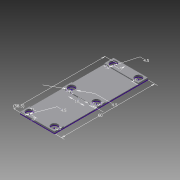
# Autodesk Inventor part: FoldLink
Saved by Autodesk Inventor 2014 SP1 (Build 180222100, 222)
## iProperties
Created: 2015-03-29
Part Number: FoldLink
Material: Generic
Document SubType Name: Modeling
Designer: Erin
Density: 1 g/cm^3
Appearance: Default
Author: Erin
Autodesk Inventor part; units mm, degrees
ref_plane "YZ Plane" through (0, 0, 0) normal (1, 0, 0) x (0, 1, 0)
ref_plane "XZ Plane" through (0, 0, 0) normal (0, 1, 0) x (-1, 0, 0)
ref_plane "XY Plane" through (0, 0, 0) normal (0, 0, 1) x (1, 0, 0)
sketch "Sketch1" plane through (0, 0, 0) normal (0, 0, 1) x (1, 0, 0)
  line L0 (-11, -30) -> (11, -30)
  line L1 (11, -30) -> (11, 30)
  line L2 (11, 30) -> (-11, 30)
  line L3 (-11, 30) -> (-11, -30)
  circle A0 centre (-8, 0) radius 2.25
  line L4 (-5, 30) -> (-5, -30) construction
  line L5 (5, 30) -> (5, -30) construction
  line L6 (0, 30) -> (0, -30) construction
  circle A1 centre (-8, 27) radius 2.25
  circle A2 centre (-8, -27) radius 2.25
  circle A3 centre (8, -27) radius 2.25
  circle A4 centre (8, 0) radius 2.25
  circle A5 centre (8, 27) radius 2.25
  line L7 (-11, 0) -> (11, 0) construction
  line L8 (-11, 30) -> (11, 30)
  line L9 (11, 30) -> (11, 24)
  line L10 (11, 24) -> (-11, 24)
  line L11 (-11, 24) -> (-11, 30)
  line L12 (-11, 3) -> (11, 3)
  line L13 (11, 3) -> (11, -3)
  line L14 (11, -3) -> (-11, -3)
  line L15 (-11, -3) -> (-11, 3)
  line L16 (-11, -30) -> (11, -30)
  line L17 (11, -30) -> (11, -24)
  line L18 (11, -24) -> (-11, -24)
  line L19 (-11, -24) -> (-11, -30)
  point P0 (0, 0)
  dimension "d0" = 4.5
  dimension "d1" = 3
  dimension "d2" = 3
  dimension "d3" = 10
  dimension "d4" = 60
  dimension "d5" = 4.5
  dimension "d6" = 3
  dimension "d7" = 3
  dimension "d8" = 4.5
  dimension "d9" = 3
  dimension "d10" = 3
  dimension "d11" = 3
  dimension "d14" = 58.5
  dimension "d15" = 3
  dimension "d16" = 3
  dimension "d17" = 3
  dimension "d18" = 3
  constraints: 40 end point, 9 point on line, 8 parallel, 6 centre point, 6 perpendicular, 4 horizontal, 4 midpoint, 3 symmetric about line, 1 horizontal alignment, 1 vertical alignment, 3 other
  measures "d0" diameter of A0
  measures "d1" distance from line of A0.centre L3
  measures "d2" distance from line of A0.centre L4
  measures "d3" distance between parallel lines of L4 L5
  measures "d4" distance of L0.end L2.start
  measures "d5" diameter of A1
  measures "d6" distance from line of A1.centre L2
  measures "d7" distance from line of A1.centre L3
  measures "d8" diameter of A2
  measures "d9" distance from line of A2.centre L0
  measures "d10" distance from line of A2.centre L3
  measures "d11" distance from line of A4.centre L5
  measures "d15" distance from line of A3.centre L18
  measures "d16" distance from line of A4.centre L14
  measures "d17" distance from line of A4.centre L12
  measures "d18" distance from line of A5.centre L10
extrude "Extrusion1" add sketch "Sketch1" along normal blind 0.6
extrude "Extrusion2" add sketch "Sketch1" along normal blind 1.2 contours L3 L18 L1 L0 | L3 L12 L1 L14 | L3 L2 L1 L10
body "Solid1"
